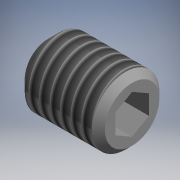
# Autodesk Inventor part: SET-SCREW8-10
Saved by Autodesk Inventor 2017.3 (Build 213256000, 256)
## iProperties
Part Number: SET-SCREW8-10
Material: Generic
Catalog Web Link: www.cadenas.de
Description: SET-SCREW-Set Screw - Flat End
Vendor: MISUMI
Document SubType Name: Modeling
Designer: partserver
Manufacturer: MISUMI
Mass: 0.431739 g
Surface Area: 3.62878 cm^2
Volume: 0.431739 cm^3
Density: 1 g/cm^3
Appearance: PSOLRGB-175-175-175
Category: PARTsolutions
Company: MISUMI
Title: SET-SCREW8-10
Author: Cadenas PARTsolutions
Comments: Set Screw - Flat End
PSOL_IDENT_0: {$CADENAS_DATA\23d-libs\misumi\metric\accessories\set_screw.prj},171 {VTYP=3D},{NB=SET-SCREW8-10},{L
PSOL_IDENT_1: INA=SET-SCREW8-10},{NN=SET-SCREW},{DATE=30.10.2020 15:47:10},{GEOMDATE=11.12.2013 00:00:00},{VERSION=
PSOL_IDENT_2: },{LINEID=60},{WBVAR=L},{WBNUMERIC=L}  {NB=SET-SCREW8-10},{LINA=SET-SCREW8-10},{KT=DUMMY},{PN=SET-SC
PSOL_IDENT_3: REW8-10},{TYPE=SET-SCREW},{M=8.0},{P=1.25},{L=10},{LMIN=4.2},{LALG=[4.2:42/0.1]},{B=4.0},{C=3.0},{DD=
PSOL_IDENT_4: 5.5}
NB: SET-SCREW8-10
NN: SET-SCREW
NT: Set Screw - Flat End
NBSYN: $PN.
LINA: SET-SCREW8-10
CATALOG: Misumi
PN: SET-SCREW8-10
M: 8
P: 1.25
L: 10
B: 4
C: 3
DD: 5.5
SUPPLIER: MISUMI
ARTICLENO: SET-SCREW8-10
BOMINFO: SET-SCREW8-10
CREATOR: CADENAS GmbH
Autodesk Inventor part; units mm, degrees
sketch "Sketch_1" plane through (0, 0, 0) normal (0, 0, 1) x (1, 0, 0)
  line L0 (0, 0) -> (-10, 0)
  line L1 (-10, 0) -> (-10, 3.233)
  line L2 (-10, 3.233) -> (-9.233, 4)
  line L3 (-9.233, 4) -> (-1.25, 4)
  line L4 (-1.25, 4) -> (0, 2.75)
  line L5 (0, 2.75) -> (0, 0)
  line L6 (0, 0) -> (-10, 0)
  constraints: 14 end point
revolve "Revolution1" add sketch "Sketch_1" angle 360 about axis through (0, 0, 0) along (1, 0, 0)
thread "Thread1" size "M8x1.25" class "6g" standard "ISO Metric profile" full length
sketch "Sketch_2" plane through (-10, 0, 0) normal (-1, 0, 0) x (0, 1, 0)
  line L0 (-2, -1.1547) -> (0, -2.3094)
  line L1 (0, -2.3094) -> (2, -1.1547)
  line L2 (2, -1.1547) -> (2, 1.1547)
  line L3 (2, 1.1547) -> (0, 2.3094)
  line L4 (0, 2.3094) -> (-2, 1.1547)
  line L5 (-2, 1.1547) -> (-2, -1.1547)
  constraints: 12 end point
extrude "Extrusion1" cut sketch "Sketch_2" against normal blind 3
sketch "Sketch_3" plane through (0, 0, 0) normal (0, 0, 1) x (1, 0, 0)
  line L0 (-5.8453, 0) -> (-7, 0)
  line L1 (-7, 0) -> (-7, 2)
  line L2 (-7, 2) -> (-5.8453, 0)
  line L3 (-5.8453, 0) -> (-7, 0)
  constraints: 8 end point
revolve "Revolution2" cut sketch "Sketch_3" angle 360 about axis through (-5.8453, 0, 0) along (1, 0, 0)
ref_plane "CP_XY" through (0, 0, 0) normal (1, 0, 0) x (0, 0, -1)
ref_plane "CP_YZ" through (0, 0, 0) normal (0, 0, -1) x (0, 1, 0)
ref_plane "CP_ZX" through (0, 0, 0) normal (0, 1, 0) x (1, 0, 0)
body "Solid1"
